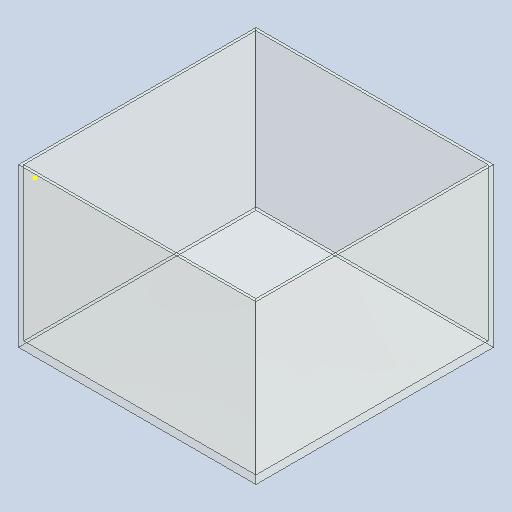
# Autodesk Inventor part: rectangle box
Saved by Autodesk Inventor 2024 (Build 280153000, 153)
## iProperties
Created: 2023-06-03
Part Number: rectangle box
Material: Glass
Document SubType Name: Modeling
Designer: Sahil Nadaf
Density: 2.18 g/cm^3
Appearance: Clear
Author: Sahil Nadaf
Autodesk Inventor part; units mm, degrees
ref_plane "YZ Plane" through (0, 0, 0) normal (1, 0, 0) x (0, 1, 0)
ref_plane "XZ Plane" through (0, 0, 0) normal (0, 1, 0) x (-1, 0, 0)
ref_plane "XY Plane" through (0, 0, 0) normal (0, 0, 1) x (1, 0, 0)
sketch "Sketch1" plane through (0, 0, 0) normal (0, 0, 1) x (1, 0, 0)
  line L0 (-25.7967, 11.5978) -> (431.4033, 11.5978)
  line L1 (431.4033, 11.5978) -> (431.4033, -293.2022)
  line L2 (431.4033, -293.2022) -> (-25.7967, -293.2022)
  line L3 (-25.7967, -293.2022) -> (-25.7967, 11.5978)
  point P0 (0, 0)
  dimension "d0" = 457.2
  dimension "d1" = 304.8
  constraints: 8 end point, 2 parallel, 1 horizontal, 1 perpendicular
  measures "d0" distance of L1.end L2.end
  measures "d1" distance of L0.end L1.end
extrude "Extrusion1" add sketch "Sketch1" along normal blind 457.2
sketch "Sketch2" plane through (-25.7967, 11.5978, 0) normal (0, 1, 0) x (1, 0, 0)
  line L0 (0, 0) -> (0, -457.2) projected
  line L1 (0, -457.2) -> (0, -452.2)
  line L2 (0, -457.2) -> (457.2, -457.2) projected
  line L3 (0, -457.2) -> (5, -457.2)
  line L4 (5, -452.2) -> (452, -452.2)
  line L5 (452, -452.2) -> (452, -5.2)
  line L6 (452, -5.2) -> (5, -5.2)
  line L7 (452, -5.2) -> (899, -5.2) construction
  line L8 (5, -452.2) -> (5, -5.2)
  point P0 (25.7967, 0)
  dimension "d4" = 5
  dimension "d5" = 5
  dimension "d6" = 447
  dimension "d7" = 447
  dimension "d8" = 447
  dimension "d9" = 180
  constraints: 14 end point, 3 horizontal, 2 point on line, 1 collinear, 1 vertical
  measures "d4" distance of L0.end L1.end
  measures "d5" distance of L0.end L3.end
  measures "d6" distance of L4.start L4.end
  measures "d7" distance of L4.end L5.end
  measures "d8" distance of L5.end L6.end
  measures "d9" angle of L6 L7
extrude "Extrusion2" cut sketch "Sketch2" against normal blind 294
sketch "Sketch3" plane through (426.2033, 11.5978, 452.2) normal (0, 0, -1) x (-1, 0, 0)
  point P0 (426.2033, -11.5978)
body "Solid1"
